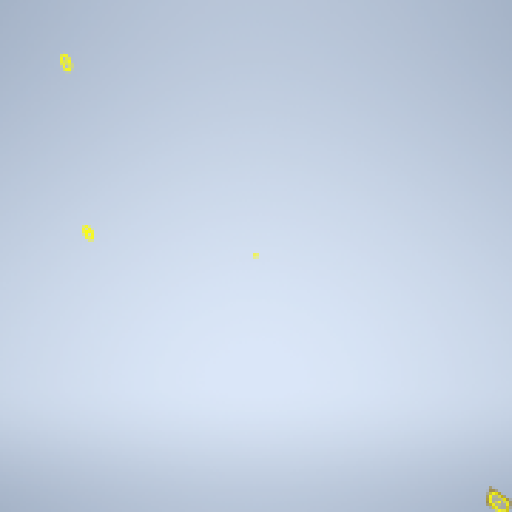
# Autodesk Inventor part: Part62
Saved by Autodesk Inventor 2023 (Build 270158000, 158)
## iProperties
Created: 2023-02-13
Part Number: Part62
Material: Generic
Document SubType Name: Modeling
Designer: klebe
Density: 1 g/cm^3
Appearance: Default
Author: klebe
Autodesk Inventor part; units mm, degrees
ref_plane "YZ Plane" through (0, 0, 0) normal (1, 0, 0) x (0, 1, 0)
ref_plane "XZ Plane" through (0, 0, 0) normal (0, 1, 0) x (-1, 0, 0)
ref_plane "XY Plane" through (0, 0, 0) normal (0, 0, 1) x (1, 0, 0)
ref_plane "Work Plane1" through (750, -285, 10) normal (0, 0, 1) x (1, 0, 0)
sketch "Sketch1" plane through (750, -285, 10) normal (0, 0, 1) x (1, 0, 0)
  circle A0 centre (0, 570) radius 23 projected
  circle A1 centre (0, 0) radius 23 projected
  circle A2 centre (-1500, 0) radius 23 projected
  circle A3 centre (-1500, 570) radius 23 projected
  point P0 (-750, 285)
extrude "Extrusion1" add sketch "Sketch1" along normal blind 500
body "Solid1"
